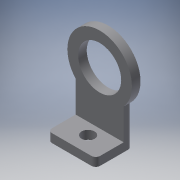
# Autodesk Inventor part: SyringeTailConnector
Saved by Autodesk Inventor 2016 (Build 200138000, 138)
## iProperties
Created: 2017-03-10
Part Number: SyringeTailConnector
Material: Generic
Document SubType Name: Modeling
Designer: Owner
Density: 1 g/cm^3
Appearance: Default
Author: Owner
Autodesk Inventor part; units mm, degrees
ref_plane "YZ Plane" through (0, 0, 0) normal (1, 0, 0) x (0, 1, 0)
ref_plane "XZ Plane" through (0, 0, 0) normal (0, 1, 0) x (-1, 0, 0)
ref_plane "XY Plane" through (0, 0, 0) normal (0, 0, 1) x (1, 0, 0)
sketch "Sketch1" plane through (0, 0, 0) normal (0, 0, 1) x (1, 0, 0)
  circle A0 centre (0, 0) radius 4.85 projected
  circle A1 centre (0, 0) radius 5
  circle A2 centre (0, 0) radius 7.5
  dimension "d0" = 10
  dimension "d1" = 15
  constraints: 2 centre point, 2 coincident
  measures "d0" diameter of A1
  measures "d1" diameter of A2
extrude "Extrusion1" add sketch "Sketch1" along normal mid plane 2 contours A2
sketch "Sketch2" plane through (0, 0, 1) normal (0, 0, 1) x (1, 0, 0)
  circle A0 centre (0, 0) radius 7.5 projected
  line L0 (-5.5902, -5) -> (0, -5)
  line L1 (0, -5) -> (0, -7.5)
  line L2 (-5.5902, -7.5) -> (-5.5902, -5)
  circle A1 centre (0, 0) radius 7.5
  line L3 (5.5902, -5) -> (0, -5)
  line L4 (5.5902, -7.5) -> (5.5902, -5)
  line L5 (3.3913, -9.725) -> (-18.205, -9.725) projected
  line L6 (-5.5902, -7.5) -> (-5.5902, -9.725)
  line L7 (5.5902, -9.725) -> (5.5902, -7.5)
  line L8 (5.5902, -9.725) -> (5.5902, -12.225)
  line L9 (5.5902, -12.225) -> (-5.5902, -12.225)
  line L10 (-5.5902, -12.225) -> (-5.5902, -9.725)
  dimension "d13" = 2.5
  constraints: 20 end point, 4 point on circle, 3 parallel, 2 symmetric about line, 1 centre point, 1 horizontal, 1 perpendicular, 1 point on line, 1 other
  measures "d13" distance of L7.start L8.end
extrude "Extrusion2" add sketch "Sketch2" against normal blind 2 contours A0 L4 L7 L8 L9 L10 L6 L2 | A0 L1 L3
sketch "Sketch5" plane through (-5.5902, -12.225, 1) normal (0, -1, 0) x (1, 0, 0)
  line L0 (11.1803, -2) -> (11.1803, 6.5)
  line L1 (11.1803, 6.5) -> (0, 6.5)
  line L2 (0, 6.5) -> (0, -2)
  line L3 (0, -2) -> (11.1803, -2)
  line L4 (11.1803, -2) -> (11.1803, 6.5)
  point P0 (5.5902, -1)
  dimension "d14" = 8.5
  constraints: 10 end point, 2 parallel, 1 horizontal, 1 perpendicular, 1 vertical
  measures "d14" distance of L0.start L0.end
extrude "Extrusion5" add sketch "Sketch5" along normal blind 2
sketch "Sketch6" plane through (-5.5902, -14.225, 1) normal (0, -1, 0) x (1, 0, 0)
  line L0 (11.1803, 6.5) -> (0, 6.5) projected
  line L1 (5.5902, 6.5) -> (5.5902, 2.69)
  circle A0 centre (5.5902, 2.69) radius 1.5
  point P0 (5.5902, -1)
  dimension "d17" = 3.81
  dimension "d18" = 3
  constraints: 2 end point, 1 centre point, 1 coincident, 1 midpoint, 1 vertical
  measures "d17" distance of L1.start L1.end
  measures "d18" diameter of A0
extrude "Extrusion6" cut sketch "Sketch6" against normal blind 2
fillet "Fillet1" radius 1 4 edges at (5.5902, -13.225, 7.5) (-5.5902, -13.225, 7.5) (5.5902, -9.6125, -1) (-5.5902, -9.6125, -1)
body "Solid1"
